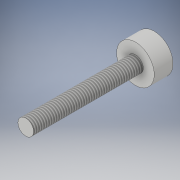
# Autodesk Inventor part: M5x30mm
Saved by Autodesk Inventor 2018 (Build 220112000, 112)
## iProperties
Created: 2017-10-07
Part Number: M5x30mm
Material: Generic
Document SubType Name: Modeling
Designer: Jurjen
Density: 1 g/cm^3
Appearance: Default
Author: Jurjen
Autodesk Inventor part; units mm, degrees
ref_plane "YZ Plane" through (0, 0, 0) normal (1, 0, 0) x (0, 1, 0)
ref_plane "XZ Plane" through (0, 0, 0) normal (0, 1, 0) x (-1, 0, 0)
ref_plane "XY Plane" through (0, 0, 0) normal (0, 0, 1) x (1, 0, 0)
sketch "Sketch1" plane through (0, 0, 0) normal (0, 1, 0) x (-1, 0, 0)
  line L0 (0, 20.5) -> (2.5, 20.5)
  line L1 (2.5, 20.5) -> (2.5, -14.5)
  line L2 (2.5, -14.5) -> (6, -14.5)
  line L3 (6, -14.5) -> (6, -20.5)
  line L4 (6, -20.5) -> (0, -20.5)
  line L5 (0, -20.5) -> (0, 20.5)
  point P0 (0, 0)
  point P1 (0, 0)
  dimension "d0" = 2.5
  dimension "d1" = 35
  dimension "d2" = 6
  dimension "d3" = 6
  constraints: 12 end point, 5 perpendicular, 1 coincident, 1 horizontal, 1 midpoint, 1 vertical alignment
  measures "d0" distance of L0.start L0.end
  measures "d1" distance of L0.end L1.end
  measures "d2" distance of L2.end L3.end
  measures "d3" distance of L3.end L4.end
revolve "Revolution1" add sketch "Sketch1" angle 360 about axis through (0, 0, -20.5) along (0, 0, 1)
thread "Thread1" size "M5x0.8" class "6g" standard "ANSI Metric M Profile" full length
body "Solid1"
